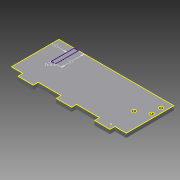
# Autodesk Inventor part: subframe
Saved by Autodesk Inventor 2014 (Build 180170000, 170)
## iProperties
Created: 2015-05-07
Part Number: subframe
Material: Generic
Document SubType Name: Modeling
Designer: cruiser
Density: 1 g/cm^3
Appearance: Default
Author: cruiser
Autodesk Inventor part; units mm, degrees
ref_plane "YZ Plane" through (0, 0, 0) normal (1, 0, 0) x (0, 1, 0)
ref_plane "XZ Plane" through (0, 0, 0) normal (0, 1, 0) x (-1, 0, 0)
ref_plane "XY Plane" through (0, 0, 0) normal (0, 0, 1) x (1, 0, 0)
sketch "Sketch1" plane through (0, 0, 0) normal (0, 0, 1) x (1, 0, 0)
  line L0 (0, 0) -> (-130, 0)
  line L1 (-130, 0) -> (-130, 62)
  line L2 (-130, 62) -> (0, 62)
  line L3 (0, 62) -> (0, 32.5)
  line L4 (0, 0) -> (20, 0)
  line L5 (20, 0) -> (20, 62)
  line L6 (20, 62) -> (0, 62)
  line L7 (0, 62) -> (0, 0)
  circle A0 centre (0, 30) radius 2.5
  circle A1 centre (14.5, 38.5) radius 2.5
  circle A2 centre (14.5, 51) radius 2.5
  line L8 (14.5, 51) -> (-130, 51)
  line L9 (-115, 0) -> (-95, 0)
  line L10 (-95, 0) -> (-95, -6.4)
  line L11 (-95, -6.4) -> (-115, -6.4)
  line L12 (-115, -6.4) -> (-115, 0)
  line L13 (-65, 0) -> (-45, 0)
  line L14 (-45, 0) -> (-45, -6.4)
  line L15 (-45, -6.4) -> (-65, -6.4)
  line L16 (-65, -6.4) -> (-65, 0)
  line L17 (-15, 0) -> (5, 0)
  line L18 (5, 0) -> (5, -6.4)
  line L19 (5, -6.4) -> (-15, -6.4)
  line L20 (-15, -6.4) -> (-15, 0)
  line L21 (-55, 62) -> (-55, 0)
  line L22 (0, 32.5) -> (0, 27.5)
  line L23 (0, 27.5) -> (0, 0)
  dimension "d0" = 20
  dimension "d1" = 150
  dimension "d2" = 62
  dimension "d3" = 5
  dimension "d4" = 5
  dimension "d5" = 5
  dimension "d6" = 30
  dimension "d7" = 14.5
  dimension "d8" = 8.5
  dimension "d9" = 12.5
  dimension "d10" = 0
  dimension "d11" = 20
  dimension "d12" = 6.4
  dimension "d15" = 50
  dimension "d20" = 75
  constraints: 48 end point, 8 parallel, 5 perpendicular, 5 point on line, 4 horizontal, 3 centre point, 2 point on circle, 1 collinear, 17 other
  measures "d0" distance of L5.end L6.end
  measures "d1" distance between parallel lines of L5 L1
  measures "d2" distance of L0.end L1.end
  measures "d3" diameter of A0
  measures "d4" diameter of A1
  measures "d5" diameter of A2
  measures "d6" distance from line of L0 A0.centre
  measures "d7" distance from line of L3 A1.centre
  measures "d8" vertical distance of A0.centre A1.centre
  measures "d9" distance of A1.centre L8.start
  measures "d10" horizontal distance of A1.centre L8.start
  measures "d11" distance of L10.end L11.end
  measures "d12" distance of L11.end L9.start
  measures "d15" distance of L9.end L14.start
  measures "d20" distance between parallel lines of L1 L21
extrude "Extrusion1" add sketch "Sketch1" along normal blind 5.6 contours L4 L18 L19 L20 L0 | L7 A0 L3 L6 L5 L4 | L0 L21 L8 L3 A0 L7 | L14 L15 L16 L0 | L0 L1 L8 L21 | L8 L21 L2 L3 | L8 L1 L2 L21 | L10 L11 L12 L0
sketch "Sketch3" plane through (0, 0, 5.6) normal (0, 0, 1) x (1, 0, 0)
  circle A0 centre (14.5, 51) radius 2.5 projected
  circle A1 centre (14.5, 38.5) radius 2.5 projected
  circle A2 centre (0, 30) radius 2.5 projected
  line L0 (-115, 0) -> (-115, -6.4) projected
  line L1 (-115, -6.4) -> (-95, -6.4) projected
  line L2 (-95, -6.4) -> (-95, 0) projected
  line L3 (-95, 0) -> (-65, 0) projected
  line L4 (-65, 0) -> (-65, -6.4) projected
  line L5 (-65, -6.4) -> (-45, -6.4) projected
  line L6 (-45, -6.4) -> (-45, 0) projected
  line L7 (-45, 0) -> (-15, 0) projected
  line L8 (-15, 0) -> (-15, -6.4) projected
  line L9 (-15, -6.4) -> (5, -6.4) projected
  line L10 (5, -6.4) -> (5, 0) projected
  line L11 (5, 0) -> (20, 0) projected
  line L12 (20, 0) -> (20, 62) projected
  line L13 (20, 62) -> (-130, 62) projected
  line L14 (-130, 62) -> (-130, 0) projected
  line L15 (-130, 0) -> (-115, 0) projected
  line L16 (-110, 62) -> (-104.4, 62)
  line L17 (-104.4, 62) -> (-104.4, 32)
  line L18 (-104.4, 32) -> (-110, 32)
  line L19 (-110, 32) -> (-110, 62)
  point P0 (0, 0)
  dimension "d33" = 5.6
  dimension "d34" = 20
  dimension "d35" = 30
  constraints: 8 end point, 2 parallel, 1 horizontal, 1 perpendicular, 1 point on line
  measures "d33" distance of L17.end L18.end
  measures "d34" distance between parallel lines of L14 L19
  measures "d35" distance of L16.end L17.end
sketch "Sketch2" plane through (0, 0, 5.6) normal (0, 0, 1) x (1, 0, 0)
  circle A0 centre (14.5, 51) radius 2.5 projected
  line L0 (20, 62) -> (-130, 62) projected
  line L1 (-130, 62) -> (-130, 0) projected
  line L2 (-110, 62) -> (-104.4, 62)
  line L3 (-104.4, 62) -> (-104.4, 51)
  line L4 (-104.4, 51) -> (-110, 51)
  line L5 (-110, 51) -> (-110, 62)
  circle A1 centre (-107.2, 41) radius 1.65
  line L6 (-107.2, 62) -> (-107.2, 51)
  arc A2 (-109.5, 51) -> (-110, 51.5) centre (-110, 51) ccw
  arc A3 (-104.4, 51.5) -> (-104.9, 51) centre (-104.4, 51) ccw
  arc A4 (-104.9, 51) -> (-104.4, 51.5) centre (-104.4, 51) ccw
  arc A5 (-110, 51.5) -> (-109.5, 51) centre (-110, 51) ccw
  point P0 (0, 0)
  dimension "d23" = 5.6
  dimension "d24" = 20
  dimension "d25" = 0
  dimension "d26" = 3.3
  dimension "d27" = 0
  dimension "d28" = 10
  dimension "d31" = 1
  dimension "d32" = 1
  constraints: 10 end point, 8 point on circle, 5 centre point, 5 point on line, 2 coincident, 2 midpoint, 2 parallel, 1 horizontal, 1 perpendicular
  measures "d23" distance of L3.end L4.end
  measures "d24" distance between parallel lines of L1 L5
  measures "d25" distance from line of A0.centre L4
  measures "d26" diameter of A1
  measures "d27" distance from line of L6 A1.centre
  measures "d28" distance from line of L4 A1.centre
  measures "d31" diameter of A2
  measures "d32" diameter of A3
equation "\"d1\" = subframe_x"
equation "\"d2\" = subframe_z"
equation "\"d12\" = wood_thickness"
equation "\"d15\" = 0.333333 * subframe_x"
equation "\"d20\" = 0.5 * subframe_x"
equation "\"t_subframe\" = thick_acrylic"
equation "\"d33\" = t_subframe"
equation "\"d23\" = t_subframe"
equation "\"wood_thickness\" = 6.4"
equation "\"m3_diameter\" = 3.15"
equation "\"m5_diameter\" = 5.25"
equation "\"stepper_screw_space\" = 35"
equation "\"stepper_shaft_diameter\" = 5"
equation "\"stepper_body_diameter\" = 28"
equation "\"laser_body_diameter\" = 12"
equation "\"thick_acrylic\" = 5.6"
equation "\"carrier_z\" = 258.6"
equation "\"carrier_z2\" = 283.6"
equation "\"thin_acrylic\" = 3"
equation "\"clear_acrylic\" = 2"
equation "\"linear_bearing_spacing\" = 216"
equation "\"linear_bearing_z\" = 304.8"
equation "\"threaded_rod_z\" = 203.2"
equation "\"motor_spacing\" = 296"
equation "\"tray_boarder\" = 15"
equation "\"bed_clamp_border\" = 15"
equation "\"brass_insert_drill\" = 4"
equation "\"brass_keep_out\" = 8"
equation "\"tape_keep_out\" = 2"
equation "\"tape_thickness\" = 2"
equation "\"crane_x\" = 245.2"
equation "\"crane_z\" = 25"
equation "\"z_min_from_center\" = 72.6"
equation "\"frame_tilt\" = 1deg"
equation "\"printer_z\" = 289"
equation "\"subframe_x\" = 150"
equation "\"subframe_z\" = 62"
body "Solid1"
